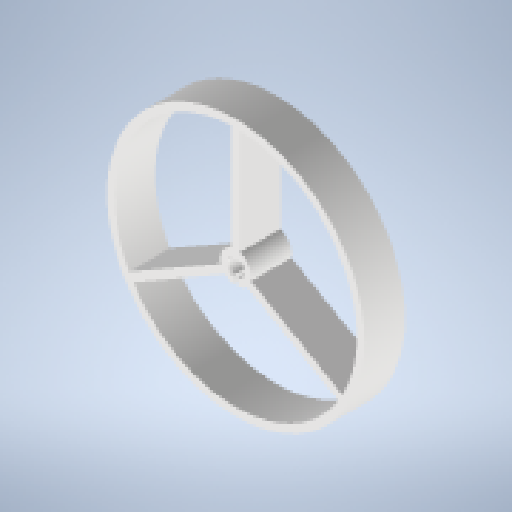
# Autodesk Inventor part: D-Shaft_Wheel3
Saved by Autodesk Inventor 2025.3 (Build 293356000, 356)
## iProperties
Created: 2025-05-20
Part Number: D-Shaft_Wheel3
Material: 一般
Document SubType Name: Modeling
Designer: yamashita1
Density: 1 g/cm^3
Appearance: 既定
Author: yamashita1
Autodesk Inventor part; units mm, degrees
ref_plane "YZ Plane" through (0, 0, 0) normal (1, 0, 0) x (0, 1, 0)
ref_plane "XZ Plane" through (0, 0, 0) normal (0, 1, 0) x (-1, 0, 0)
ref_plane "XY Plane" through (0, 0, 0) normal (0, 0, 1) x (1, 0, 0)
sketch "スケッチ1" plane through (0, 0, 0) normal (0, 0, 1) x (1, 0, 0)
  circle A0 centre (0, 0) radius 1.5
  circle A1 centre (0, 0) radius 3.1
  line L0 (-0.4, 0) -> (0.4, 0)
  line L1 (0.4, 0) -> (0.4, -3.1)
  line L2 (0.4, -3.1) -> (-0.4, -3.1)
  line L3 (-0.4, -3.1) -> (-0.4, 0)
  line L4 (-1.0712, 1.05) -> (1.0712, 1.05)
  circle A2 centre (0, 0) radius 25.5
  circle A3 centre (0, 0) radius 23.9
  line L5 (-1.4605, 1.0815) -> (-1.1105, 1.4385)
  line L6 (-1.1105, 1.4385) -> (0.175, 0.1785)
  line L7 (0.175, 0.1785) -> (-0.175, -0.1785)
  line L8 (-0.175, -0.1785) -> (-1.4605, 1.0815)
  line L9 (1.4605, 1.0815) -> (1.1105, 1.4385)
  line L10 (1.1105, 1.4385) -> (-0.175, 0.1785)
  line L11 (-0.175, 0.1785) -> (0.175, -0.1785)
  line L12 (0.175, -0.1785) -> (1.4605, 1.0815)
  line L13 (0, 0) -> (-1.0712, 1.05) construction
  line L14 (1.0712, 1.05) -> (0, 0) construction
  point P0 (0.4, -1.4457)
  point P1 (0.4, -3.0741)
  point P2 (-0.4, -3.0741)
  point P3 (-0.4, -1.4457)
  point P4 (-0.7141, 1.05)
  point P5 (0.7141, 1.05)
  point P6 (1.2312, 0.8568)
  point P7 (-1.2312, 0.8568)
  dimension "SHAFT_D" = 3
  dimension "SLIT" = 0.8
  dimension "HUB_THIN" = 1.6
  dimension "d3" = 1.05
  dimension "WHEEL_D" = 51
  dimension "d5" = 1.6
  dimension "d18" = 0.5
  dimension "d19" = 1.8
  constraints: 30 end point, 8 parallel, 5 coincident, 4 centre point, 3 midpoint, 3 perpendicular, 2 equal length, 2 horizontal, 2 point on circle, 1 tangent
  measures "SHAFT_D" diameter of A0
  measures "SLIT" distance between parallel lines of L1 L3
  measures "HUB_THIN" radial gap between concentric circles of A1 A0
  measures "d3" distance from line of L4 A0.centre
  measures "WHEEL_D" diameter of A2
  measures "d5" radial gap between concentric circles of A2 A3
  measures "d18" distance between parallel lines of L10 L12
  measures "d19" distance of L11.end L9.start
extrude "ハブ＆リム" add sketch "スケッチ1" along normal blind 8 contours A0 L12 L9 L10 L6 L5 L8 L3 A1 L1 | L10 L4 L6 A0 | A2
sketch "スケッチ2" plane through (0, 0, 0) normal (0, 0, 1) x (1, 0, 0)
  line L0 (-0.8, 2.6) -> (0.8, 2.6)
  line L1 (0.8, 2.6) -> (0.8, 23.9)
  line L2 (0.8, 23.9) -> (-0.8, 23.9)
  line L3 (-0.8, 23.9) -> (-0.8, 2.6)
  circle A0 centre (0, 0) radius 23.9 projected
  point P0 (0, 23.9)
  dimension "d8" = 1.6
  dimension "d9" = 2.6
  constraints: 8 end point, 2 parallel, 1 horizontal, 1 midpoint, 1 perpendicular, 1 tangent, 1 vertical alignment
  measures "d8" distance between parallel lines of L1 L3
  measures "d9" distance from line of point (0, 0) L0
extrude "スポーク" add sketch "スケッチ2" along normal up to surface (8 mm away) contours L3 A0 L1 L0 | L3 L2 A0 | A0 L2 L1 picked at (0, 9.7)
pattern_circular "円形状パターン1" count 3 over 360 about axis through (0, 0, -10) along (0, 0, 1) of "スポーク"
chamfer "面取り1" distance 0.3 angle 45 3 edges at (-1.4109, -0.5094, 8) (0, 1.05, 8) (1.4109, -0.5094, 8)
equation "\"d5\" = HUB_THIN"
